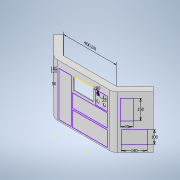
# Autodesk Inventor part: MAIN CONTROLLER
Saved by Autodesk Inventor 2020 (Build 240168000, 168)
## iProperties
Created: 2020-04-01
Part Number: MAIN CONTROLLER
Material: Generic
Document SubType Name: Modeling
Designer: Yusuf
Density: 1 g/cm^3
Appearance: Default
Author: Yusuf
Autodesk Inventor part; units mm, degrees
ref_plane "YZ Plane" through (0, 0, 0) normal (1, 0, 0) x (0, 1, 0)
ref_plane "XZ Plane" through (0, 0, 0) normal (0, 1, 0) x (-1, 0, 0)
ref_plane "XY Plane" through (0, 0, 0) normal (0, 0, 1) x (1, 0, 0)
sketch "Sketch1" plane through (0, 0, 0) normal (0, 1, 0) x (-1, 0, 0)
  line L0 (-25, 400) -> (25, 400)
  line L1 (25, 400) -> (25, -400)
  line L2 (25, -400) -> (-25, -400)
  line L3 (-25, -400) -> (-25, 400)
  line L4 (-25, 400) -> (25, -400) construction
  line L5 (25, 400) -> (-25, -400) construction
  line L6 (25, 0) -> (-25, 0)
  line L7 (-25, 0) -> (-25, -200)
  line L8 (-25, -200) -> (25, -200)
  line L9 (25, -200) -> (25, 0)
  line L10 (25, 0) -> (-25, 0)
  line L11 (-25, 0) -> (-25, 200)
  line L12 (-25, 200) -> (25, 200)
  line L13 (25, 200) -> (25, 0)
  point P0 (0, 0)
  dimension "d0" = 50
  dimension "d1" = 800
  dimension "d2" = 200
  dimension "d3" = 200
  constraints: 28 end point, 6 parallel, 3 horizontal, 3 midpoint, 3 perpendicular, 2 point on line
  measures "d0" distance of L1.end L2.end
  measures "d1" distance of L0.end L1.end
  measures "d2" distance of L7.end L6.end
  measures "d3" distance of L10.end L11.end
extrude "Extrusion1" add sketch "Sketch1" along normal blind 400
sketch "Sketch4" plane through (25, 0, 400) normal (1, 0, 0) x (0, 0, -1)
  line L0 (0, 0) -> (800, 0) projected
  line L1 (800, 0) -> (800, 400) projected
  line L2 (0, 400) -> (800, 400) projected
  line L3 (0, 0) -> (0, 400) projected
  line L4 (0, 400) -> (800, 400) projected
  line L5 (200, 400) -> (200, 0)
  line L6 (0, 0) -> (800, 0) projected
  line L7 (600, 400) -> (600, 0)
  point P0 (400, 0)
  dimension "d6" = 200
  dimension "d7" = 200
  constraints: 4 end point, 4 point on line, 2 perpendicular
  measures "d6" distance between parallel lines of L3 L5
  measures "d7" distance between parallel lines of L1 L7
bend part "Bend Part1" radius 10 angle 45 line through (25, 400, 200) along (0, -1, 0) centre toward (1, 0, 0) moving side (0, 0, 1) both sides no
bend part "Bend Part2" radius 10 angle 45 line through (25, 400, -200) along (0, -1, 0) centre toward (1, 0, 0) moving side (0, 0, -1) both sides no
shell "Shell1" thickness 5 removed faces 3 at (25, 133.3333, 66.6667) at (73.2182, 133.3333, -252.3603) at (118.5074, 133.3333, 297.6496)
sketch "Sketch5" plane through (-25, 0, -200) normal (-1, 0, 0) x (0, 0, 1)
  line L0 (125, 350) -> (275, 350)
  line L1 (275, 350) -> (275, 260)
  line L2 (275, 260) -> (125, 260)
  line L3 (125, 260) -> (125, 350)
  line L4 (0, 0) -> (400, 0) projected
  point P0 (200, 0)
  point P1 (200, 350)
  dimension "d13" = 90
  dimension "d14" = 150
  dimension "d15" = 260
  constraints: 8 end point, 2 parallel, 1 horizontal, 1 midpoint, 1 perpendicular
  measures "d13" distance of L0.end L1.end
  measures "d14" distance of L1.end L2.end
  measures "d15" distance between parallel lines of L4 L2
extrude "Extrusion2" cut sketch "Sketch5" against normal through all
sketch "Sketch6" plane through (-25, 0, -200) normal (-1, 0, 0) x (0, 0, 1)
  line L0 (12.5071, 349.8545) -> (104.9693, 349.8545)
  line L1 (104.9693, 349.8545) -> (104.9693, 11.9858)
  line L2 (104.9693, 11.9858) -> (12.5071, 11.9858)
  line L3 (12.5071, 11.9858) -> (12.5071, 349.8545)
  line L4 (114.3868, 240.5731) -> (380.6439, 240.5731)
  line L5 (380.6439, 240.5731) -> (380.6439, 139.5495)
  line L6 (380.6439, 139.5495) -> (114.3868, 139.5495)
  line L7 (114.3868, 139.5495) -> (114.3868, 240.5731)
  line L8 (114.3868, 127.6438) -> (380.6439, 127.6438)
  line L9 (380.6439, 127.6438) -> (380.6439, 11.9858)
  line L10 (380.6439, 11.9858) -> (114.3868, 11.9858)
  line L11 (114.3868, 11.9858) -> (114.3868, 127.6438)
  line L12 (125, 350) -> (275, 350) projected
  line L13 (290.5216, 350) -> (380.6439, 350)
  line L14 (380.6439, 350) -> (380.6439, 248.5458)
  line L15 (380.6439, 248.5458) -> (290.5216, 248.5458)
  line L16 (290.5216, 248.5458) -> (290.5216, 350)
  circle A0 centre (310.5216, 330) radius 11
  point P0 (200, 0)
  dimension "d18" = 22
  dimension "d19" = 20
  dimension "d20" = 20
  constraints: 32 end point, 8 parallel, 4 horizontal, 4 perpendicular, 3 point on line, 1 centre point
  measures "d18" diameter of A0
  measures "d19" distance from line of L13 A0.centre
  measures "d20" distance from line of L16 A0.centre
extrude "Extrusion3" cut sketch "Sketch6" against normal through all contours A0
pattern_linear "Rectangular Pattern1" count 2 spacing 50 along (0, 0, 1) count 2 spacing 50 along (0, -1, 0) of "Extrusion3"
sketch "Sketch7" plane through (-7.4264, 0, -242.4264) normal (-0.7071068, 0, -0.7071068) x (-0.7071068, 0, 0.7071068)
  point P0 (166.1701, 0)
sketch "Sketch8" plane through (-7.4264, 0, -242.4264) normal (-0.7071068, 0, -0.7071068) x (-0.7071068, 0, 0.7071068)
  line L0 (-164.1941, 360.4617) -> (-44.1941, 360.4617)
  line L1 (-44.1941, 360.4617) -> (-44.1941, 260.4617)
  line L2 (-44.1941, 260.4617) -> (-164.1941, 260.4617)
  line L3 (-164.1941, 260.4617) -> (-164.1941, 360.4617)
  line L4 (-164.1941, 233.4068) -> (-44.1941, 233.4068)
  line L5 (-44.1941, 233.4068) -> (-44.1941, 183.4068)
  line L6 (-44.1941, 183.4068) -> (-164.1941, 183.4068)
  line L7 (-164.1941, 183.4068) -> (-164.1941, 233.4068)
  point P0 (166.1701, 0)
  dimension "d29" = 120
  dimension "d30" = 100
  dimension "d31" = 50
  constraints: 16 end point, 4 parallel, 2 horizontal, 2 perpendicular
  measures "d29" distance of L1.end L2.end
  measures "d30" distance of L0.end L1.end
  measures "d31" distance of L4.end L5.end
sketch "Sketch9" plane through (-7.4264, 0, 242.4264) normal (-0.7071068, 0, 0.7071068) x (0.7071068, 0, 0.7071068)
  line L0 (13.7989, 359.3191) -> (83.7989, 359.3191)
  line L1 (83.7989, 359.3191) -> (83.7989, 209.3191)
  line L2 (83.7989, 209.3191) -> (13.7989, 209.3191)
  line L3 (13.7989, 209.3191) -> (13.7989, 359.3191)
  line L4 (19.0929, 151.9727) -> (159.0929, 151.9727)
  line L5 (159.0929, 151.9727) -> (159.0929, 51.9727)
  line L6 (159.0929, 51.9727) -> (19.0929, 51.9727)
  line L7 (19.0929, 51.9727) -> (19.0929, 151.9727)
  point P0 (-166.1701, 0)
  dimension "d32" = 70
  dimension "d33" = 150
  dimension "d34" = 140
  dimension "d35" = 100
  constraints: 16 end point, 4 parallel, 2 horizontal, 2 perpendicular
  measures "d32" distance of L1.end L2.end
  measures "d33" distance of L0.end L1.end
  measures "d34" distance of L5.end L6.end
  measures "d35" distance of L4.end L5.end
body "Solid1"
